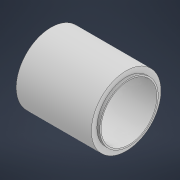
# Autodesk Inventor part: 3
Saved by Autodesk Inventor 2022 (Build 260153000, 153)
## iProperties
Created: 2022-09-05
Part Number: 3
Material: 일반
Document SubType Name: Modeling
Designer: USER
Density: 1 g/cm^3
Appearance: 기본값
Author: USER
Autodesk Inventor part; units mm, degrees
ref_plane "YZ Plane" through (0, 0, 0) normal (1, 0, 0) x (0, 1, 0)
ref_plane "XZ Plane" through (0, 0, 0) normal (0, 1, 0) x (-1, 0, 0)
ref_plane "XY Plane" through (0, 0, 0) normal (0, 0, 1) x (1, 0, 0)
sketch "스케치1" plane through (0, 0, 0) normal (0, 0, 1) x (1, 0, 0)
  line L0 (-16.8252, 0) -> (22.3466, 0)
  line L1 (-13.5, 0) -> (14.5, 0)
  line L2 (14.5, 0) -> (14.5, 10)
  line L3 (14.5, 10) -> (-13.5, 10)
  line L4 (-13.5, 10) -> (-13.5, 0)
  line L5 (-13.5, 0) -> (13.5, 0)
  line L6 (13.5, 0) -> (13.5, 12.5)
  line L7 (13.5, 12.5) -> (-13.5, 12.5)
  line L8 (-13.5, 12.5) -> (-13.5, 0)
  point P0 (0, 0)
  point P1 (13.5, 10)
  dimension "d0" = 20
  dimension "d1" = 25
  dimension "d2" = 27
  dimension "d3" = 28
  dimension "d4" = 13.5
  dimension "d5" = 13.5
  constraints: 18 end point, 4 parallel, 3 horizontal, 2 perpendicular, 2 point on line
  measures "d0" diameter of L3 L0
  measures "d1" diameter of L7 L0
  measures "d2" distance between parallel lines of L6 L8
  measures "d3" distance between parallel lines of L2 L4
  measures "d4" distance from line of L4 point (0, 0)
  measures "d5" distance from line of L8 point (0, 0)
revolve "회전1" add sketch "스케치1" angle 360 about axis through (-16.8252, 0, 0) along (1, 0, 0) contours L8 L7 L6 L3
sketch "스케치2" plane through (13.5, 0, 0) normal (1, 0, 0) x (0, 0, -1)
  circle A0 centre (0, 0) radius 10.5
  circle A1 centre (0, 0) radius 10
  dimension "d7" = 21
  dimension "d8" = 20
  constraints: 2 centre point, 2 coincident
  measures "d7" diameter of A0
  measures "d8" diameter of A1
extrude "돌출1" add sketch "스케치2" along normal blind 1
